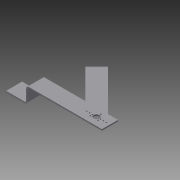
# Autodesk Inventor part: Encoder Mounting
Saved by Autodesk Inventor 2013 (Build 170138000, 138)
## iProperties
Created: 2013-01-28
Part Number: Encoder Mounting
Material: Generic
Document SubType Name: Sheet Metal
Designer: actoennies
Density: 1 g/cm^3
Sheet Metal Rule: Default
Author: actoennies
Autodesk Inventor part; units mm, degrees
ref_plane "YZ Plane" through (0, 0, 0) normal (1, 0, 0) x (0, 1, 0)
ref_plane "XZ Plane" through (0, 0, 0) normal (0, 1, 0) x (-1, 0, 0)
ref_plane "XY Plane" through (0, 0, 0) normal (0, 0, 1) x (1, 0, 0)
sketch "Sketch1" plane through (0, 0, 0) normal (0, 1, 0) x (-1, 0, 0)
  circle A0 centre (9.525, 0) radius 1.5875
  circle A1 centre (-9.525, 0) radius 1.5875
  circle A2 centre (9.0518, 5.2261) radius 1.5875
  circle A3 centre (0, -10.4521) radius 1.5875
  circle A4 centre (-9.0518, 5.226) radius 1.5875
  circle A5 centre (-16.256, 0) radius 1.4351
  circle A6 centre (16.256, 0) radius 1.4351
  circle A7 centre (23.0124, 0) radius 1.4351
  circle A8 centre (-23.0124, 0) radius 1.4351
  circle A9 centre (0, 0) radius 6.9532
  line L0 (-31.75, 19.05) -> (44.45, 19.05)
  line L1 (-7.8908, -19.05) -> (14.5599, -41.5006)
  line L2 (45.9908, -19.05) -> (117.8328, -90.892)
  line L3 (44.45, 19.05) -> (147.5908, 19.05)
  line L4 (45.9908, -19.05) -> (147.5908, -19.05)
  line L5 (147.5908, 19.05) -> (147.5908, -19.05)
  line L6 (117.8328, -90.892) -> (90.892, -117.8328)
  line L7 (14.5599, -41.5006) -> (90.892, -117.8328)
  line L8 (-31.75, 19.05) -> (-31.75, -19.05)
  line L9 (-31.75, -19.05) -> (-7.8908, -19.05)
  point P0 (0, 0)
  point P1 (-1.5408, -25.4)
  dimension "d5" = 76.2
  dimension "d7" = 19.05
  dimension "d34" = 38.1
  dimension "d35" = 38.1
  dimension "d36" = 19.05
  dimension "d37" = 19.05
  dimension "d39" = 45
  dimension "d41" = 101.6
  dimension "d42" = 101.6
  dimension "d43" = 19.05
  dimension "d44" = 31.75
  measures "d5" distance of L0.start L0.end
  measures "d7" distance from line of L0 point (0, 0)
  measures "d34" distance between parallel lines of L3 L4
  measures "d35" distance between parallel lines of L1 L2
  measures "d36" distance from line of point (0, 0) L1
  measures "d37" distance from line of point (0, 0) L3
  measures "d39" angle of L4 L2
  measures "d41" distance from line of L2.start L5
  measures "d42" distance of L2.start L2.end
  measures "d43" distance from line of L9 point (0, 0)
  measures "d44" distance from line of point (0, 0) L8
extrude "Plate1" add sketch "Sketch1" along normal blind 3.175
sketch "Sketch4" plane through (-88.647, 3.175, -115.5878) normal (-0.7071068, 0, -0.7071068) x (0, -1, 0)
  line L0 (0, 38.1) -> (0, 0)
  line L1 (0, 0) -> (50.8, 0)
  line L2 (50.8, 0) -> (50.8, 38.1)
  line L3 (50.8, 38.1) -> (0, 38.1)
  constraints: 6 end point, 1 horizontal, 1 perpendicular, 1 vertical
edge flange "Flange3" height 50.8 angle 90 thickness 3.175 bend radius 3.175 thickness toward (-0.7071068, 0, -0.7071068) relief straight relief width 3.175 relief depth 1.5875 corner gap 3.175 corner form 0 edges at (-104.3624, 0, -104.3624) (-147.5908, 0, 0) wall of the first edge with corners at (-115.5878, 3.175, -88.647) (-88.647, 3.175, -115.5878) (-88.647, -47.625, -115.5878) (-115.5878, -47.625, -88.647)
bend "Bend3"
corner "Corner3"
sketch "Sketch5" plane through (-115.5878, -44.45, -88.647) normal (0, -1, 0) x (1, 0, 0)
  line L0 (26.9408, -26.9408) -> (0, 0)
  line L1 (0, 0) -> (-35.921, -35.921)
  line L2 (-35.921, -35.921) -> (-8.9803, -62.8618)
  line L3 (-8.9803, -62.8618) -> (26.9408, -26.9408)
  constraints: 6 end point, 1 perpendicular, 2 other
edge flange "Flange4" height 50.8 angle 90 thickness 3.175 bend radius 3.175 thickness toward (0, -1, 0) relief straight relief width 3.175 relief depth 1.5875 corner gap 3.175 corner form 0 edges at (-104.3624, -47.625, -104.3624) (-147.5908, -47.625, 0) wall of the first edge with corners at (-88.647, -44.45, -115.5878) (-115.5878, -44.45, -88.647) (-151.5088, -44.45, -124.568) (-124.568, -44.45, -151.5088)
bend "Bend4"
corner "Corner4"
sketch "Sketch6" plane through (-195.2158, -44.45, 19.05) normal (0, 1, 0) x (1, 0, 0)
  line L0 (44.45, 0) -> (44.45, 38.1) projected
  line L1 (0, 38.1) -> (44.45, 38.1) projected
  line L2 (0, 38.1) -> (0, 0) projected
  circle A0 centre (6.35, 19.05) radius 3.3782
  circle A1 centre (38.1, 19.05) radius 3.3782
  point P0 (195.2158, 19.05)
  dimension "d65" = 6.7564
  dimension "d66" = 6.7564
  dimension "d67" = 6.35
  dimension "d68" = 19.05
  dimension "d69" = 19.05
  dimension "d70" = 6.35
  constraints: 2 centre point
  measures "d65" diameter of A0
  measures "d66" diameter of A1
  measures "d67" distance from line of L2 A0.centre
  measures "d68" distance from line of L1 A0.centre
  measures "d69" distance from line of L1 A1.centre
  measures "d70" distance from line of L0 A1.centre
extrude "Cut1" cut sketch "Sketch6" against normal blind 3.175
sketch "Sketch7" plane through (-151.5088, -44.45, -124.568) normal (0, 1, 0) x (0.7071068, 0, 0.7071068)
  line L0 (44.45, 0) -> (44.45, 38.1) projected
  line L1 (0, 38.1) -> (0, 0) projected
  line L2 (0, 0) -> (44.45, 0) projected
  circle A0 centre (6.35, 19.05) radius 3.3782
  circle A1 centre (38.1, 19.05) radius 3.3782
  point P0 (195.2158, 19.05)
  dimension "d73" = 6.7564
  dimension "d74" = 6.7564
  dimension "d75" = 6.35
  dimension "d76" = 19.05
  dimension "d77" = 19.05
  dimension "d78" = 6.35
  constraints: 2 centre point
  measures "d73" diameter of A0
  measures "d74" diameter of A1
  measures "d75" distance from line of L1 A0.centre
  measures "d76" distance from line of L2 A0.centre
  measures "d77" distance from line of L2 A1.centre
  measures "d78" distance from line of L0 A1.centre
extrude "Cut2" cut sketch "Sketch7" against normal blind 3.175
equation "\"d71\" = Thickness"
equation "\"d79\" = Thickness"
equation "\"d45\" = BendReliefWidth"
equation "\"d46\" = BendReliefDepth"
equation "\"d47\" = MinimumRemnant"
equation "\"d48\" = BendRadius"
equation "\"d51\" = BendRadius"
equation "\"d52\" = CornerReliefSize"
equation "\"d53\" = GapSize"
equation "\"d54\" = JacobiRadiusSize"
equation "\"d55\" = BendReliefWidth"
equation "\"d56\" = BendReliefDepth"
equation "\"d57\" = MinimumRemnant"
equation "\"d58\" = BendRadius"
equation "\"d61\" = BendRadius"
equation "\"d62\" = CornerReliefSize"
equation "\"d63\" = GapSize"
equation "\"d64\" = JacobiRadiusSize"
equation "\"BendRadius\" = Thickness"
equation "\"BendReliefWidth\" = Thickness"
equation "\"BendReliefDepth\" = 0.5 * Thickness"
equation "\"CornerReliefSize\" = 4 * Thickness"
equation "\"MinimumRemnant\" = 2 * Thickness"
equation "\"TransitionRadius\" = BendRadius"
equation "\"JacobiRadiusSize\" = BendRadius"
equation "\"GapSize\" = Thickness"
equation "\"d8\" = BendRadius"
equation "\"Thickness\" = 3.175"
body "Solid1"
